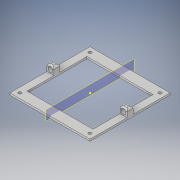
# Autodesk Inventor part: Pièce5
Saved by Autodesk Inventor 2019 (Build 230136000, 136)
## iProperties
Created: 2018-09-17
Part Number: Pièce5
Material: Generico
Document SubType Name: Modeling
Designer: acorbeau
Density: 1 g/cm^3
Appearance: Default
Author: acorbeau
Autodesk Inventor part; units mm, degrees
ref_plane "YZ Plane" through (0, 0, 0) normal (1, 0, 0) x (0, 1, 0)
ref_plane "XZ Plane" through (0, 0, 0) normal (0, 1, 0) x (-1, 0, 0)
ref_plane "XY Plane" through (0, 0, 0) normal (0, 0, 1) x (1, 0, 0)
sketch "Esquisse1" plane through (0, 0, 0) normal (0, 1, 0) x (-1, 0, 0)
  line L0 (-40, 40) -> (40, 40)
  line L1 (40, 40) -> (40, -40)
  line L2 (40, -40) -> (-40, -40)
  line L3 (-40, -40) -> (-40, 40)
  line L4 (-40, 40) -> (40, -40) construction
  line L5 (40, 40) -> (-40, -40) construction
  point P0 (0, 0)
  dimension "d0" = 80
  constraints: 12 end point, 2 midpoint, 2 parallel, 2 perpendicular, 1 horizontal
  measures "d0" distance of L0.end L1.end
extrude "Extrusion1" add sketch "Esquisse1" along normal blind 2
sketch "Esquisse2" plane through (0, 2, 0) normal (0, 1, 0) x (1, 0, 0)
  point P0 (0, 0)
sketch "Esquisse3" plane through (0, 2, 0) normal (0, 1, 0) x (1, 0, 0)
  line L0 (33, -30) -> (-33, -30)
  line L1 (-33, -30) -> (-33, 30)
  line L2 (-33, 30) -> (33, 30)
  line L3 (33, 30) -> (33, -30)
  line L4 (33, -30) -> (-33, 30) construction
  line L5 (-33, -30) -> (33, 30) construction
  point P0 (0, 0)
  dimension "d3" = 66
  dimension "d4" = 60
  constraints: 12 end point, 2 midpoint, 2 parallel, 1 horizontal, 1 perpendicular
  measures "d3" distance of L1.end L2.end
  measures "d4" distance of L0.end L1.end
extrude "Extrusion2" cut sketch "Esquisse3" against normal blind 10
sketch "Esquisse10" plane through (0, 2, 0) normal (0, 1, 0) x (1, 0, 0)
  line L0 (35, 35) -> (-35, 35)
  line L1 (-35, 35) -> (-35, -35)
  line L2 (-35, -35) -> (35, -35)
  line L3 (35, -35) -> (35, 35)
  line L4 (35, 35) -> (-35, -35) construction
  line L5 (-35, 35) -> (35, -35) construction
  line L6 (-40, 40) -> (-40, -40) projected
  line L7 (-40, -40) -> (40, -40) projected
  point P0 (0, 0)
  point P1 (-40, -5)
  dimension "d23" = 5
  dimension "d24" = 5
  constraints: 12 end point, 2 midpoint, 2 parallel, 1 horizontal, 1 perpendicular
  measures "d23" distance from line of L6 L1.end
  measures "d24" distance from line of L7 L1.end
hole "Perçage1" at (35, 2, 35) at (-35, 2, 35) at (-35, 2, -35) at (35, 2, -35) direction (0, -1, 0) diameter 3 depth 66.675 tip angle 118
sketch "Esquisse11" plane through (0, 2, 0) normal (0, 1, 0) x (1, 0, 0)
  line L0 (40, -40) -> (40, 40) projected
  line L1 (33, 30) -> (33, -30) projected
  line L2 (40, 3) -> (33, 3)
  line L3 (33, 3) -> (33, -3)
  line L4 (33, -3) -> (40, -3)
  line L5 (40, -3) -> (40, 3)
  point P0 (0, 0)
  dimension "d37" = 3
  dimension "d38" = 3
  constraints: 8 end point, 2 parallel, 2 point on line, 1 horizontal, 1 perpendicular
  measures "d37" distance from line of point (0, 0) L2
  measures "d38" distance from line of point (0, 0) L4
extrude "Extrusion9" add sketch "Esquisse11" along normal blind 7
sketch "Esquisse12" plane through (40, 2, -3) normal (0, 0, -1) x (-1, 0, 0)
  line L0 (7, 0) -> (0, 0) projected
  line L1 (0, 0) -> (7, 6.8816)
  line L2 (0, 0) -> (0, 7) projected
  line L3 (7, 0) -> (0, 7)
  point P0 (40, -2)
  point P1 (3.5, 3.5)
  constraints: 4 end point, 1 midpoint
hole "Perçage2" at (36.5, 5.5, -3) direction (0, 0, 1) diameter 5 depth 66.675 tip angle 118
fillet "Congé1" radius 2 4 edges at (36.5, 9, -3) (40, 9, 0) (36.5, 9, 3) (33, 9, 0)
ref_plane "Plan de construction1" through (0, 0, -40) normal (-1, 0, 0) x (0, 0, 1)
mirror "Symétrie1" about plane through (0, 0, -40) normal (-1, 0, 0) of "Extrusion9", "Perçage2", "Congé1"
